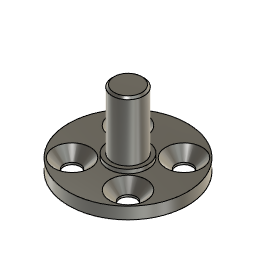
Pan axis shaft (Autodesk Fusion 360 design; units mm, degrees)
Autodesk Fusion 360 part; units mm, degrees
sketch "Szkic1" plane through (0, 0, 0) normal (0, 0, 1) x (1, 0, 0)
  circle A0 centre (0, 0) radius 15
  dimension "d1" = 30
  constraint coincident A0.centre origin
  measures "d1" diameter of A0
extrude "Wyciągnięcie proste1" add sketch "Szkic1" along normal blind 3
sketch "Szkic2" plane through (0, 0, 3) normal (0, 0, 1) x (-1, 0, 0)
  circle A0 centre (0, 0) radius 15
  circle A1 centre (0, 0) radius 4
  dimension "d4" = 8
  constraint coincident A0.centre A1.centre
  measures "d4" diameter of A1
extrude "Wyciągnięcie proste2" add sketch "Szkic2" along normal blind 16 contours A1
sketch "Szkic3" plane through (0, 0, 3) normal (0, 0, 1) x (-1, 0, 0)
  circle A0 centre (0, 0) radius 4
  circle A1 centre (0, 0) radius 15
  circle A2 centre (-10, 0) radius 2.1
  circle A3 centre (0, -10) radius 2.1
  circle A4 centre (10, 0) radius 2.1
  circle A5 centre (0, 10) radius 2.1
  dimension "d7" = 4.2
  dimension "d8" = 4.2
  dimension "d9" = 4.2
  dimension "d10" = 4.2
  measures "d7" diameter of A2
  measures "d8" diameter of A3
  measures "d9" diameter of A4
  measures "d10" diameter of A5
extrude "Wyciągnięcie proste3" cut sketch "Szkic3" against normal blind 3 contours A2 | A3 | A4 | A5
chamfer "Fazowanie1" distance 2.5 angle 45 4 edges at (11.9579, -0.7594, 3) (1.9579, -10.7594, 3) (-8.0421, -0.7594, 3) (1.9579, 9.2406, 3)
chamfer "Fazowanie2" distance 0.5 angle 45 1 edges at (3.7293, 1.4465, 19)
sketch "Szkic4" plane through (0, 0, 3) normal (0, 0, 1) x (-1, 0, 0)
  circle A0 centre (10, 0) radius 4.6
  circle A1 centre (-10, 0) radius 4.6
  circle A2 centre (0, 0) radius 4
  circle A3 centre (0, 0) radius 15
  circle A4 centre (0, 10) radius 4.6
  circle A5 centre (0, -10) radius 4.6
  circle A6 centre (0, 0) radius 5
  constraint coincident A2.centre A3.centre
extrude "Wyciągnięcie proste4" add sketch "Szkic4" along normal blind 1 contours A6
move_body "Przesuń1" bodies 1 to x (0.707107, -0.707107, 0) y (0.707107, 0.707107, 0) z (0, 0, 1) at (0, 0, 0)
sketch "Szkic5" plane through (0, 0, 0) normal (0, 1, 0) x (1, 0, 0)
